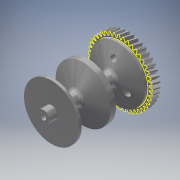
# Autodesk Inventor part: Spur Gear22
Saved by Autodesk Inventor 2019 (Build 230136000, 136)
## iProperties
Created: 2020-07-29
Part Number: Spur Gear22
Material: Steel
Document SubType Name: Modeling
Designer: Ian
Categories: <?xml version="1.0" encoding="UTF-16"?> <MemberInstance><Categories><FamilyTemplate><FamilyTemplateParameter ValueType="xs:double" Id="1" ObjectReferenceKey="da_z" ObjectType="kUserParameterObject"/><FamilyTemplateParameter ValueType="xs:double" Id="2" ObjectReferenceKey="da_b" ObjectType="kUserParameterObject"/><FamilyTemplateParameter ValueType="xs:double" Id="3" ObjectReferenceKey="da_beta" ObjectType="kUserParameterObject"/><FamilyTemplateParameter ValueType="xs:double" Id="4" ObjectReferenceKey="da_da" ObjectType="kUserParameterObject"/><FamilyTemplateParameter ValueType="xs:double" Id="5" ObjectReferenceKey="da_aw" ObjectType="kUserParameterObject"/><FamilyTemplateParameter ValueType="xs:string" Id="6" ObjectReferenceKey="EAIAABAAAACIAQAAAAAAAIAAAAAAAAAA" ObjectType="83910656" SubObjectId="SurfaceGeometry"/></FamilyTemplate><ParamToTemplateMap><ParamToTemplate CategoryParameter="//CategoryParameter[@InternalName='046C89C9-8512-4d59-83FE-43B91F4F132A']" TemplateParameter="1"/><ParamToTemplate CategoryParameter="//CategoryParameter[@InternalName='2552DF32-E462-4b46-AEBF-C6C7768E72AC']" TemplateParameter="2"/><ParamToTemplate CategoryParameter="//CategoryParameter[@InternalName='C9EE641D-15FC-4fae-A226-E94C4372FDD7']" TemplateParameter="3"/><ParamToTemplate><ParamToTemplate CategoryParameter="//CategoryParameter[@InternalName='00B6519A-459B-49c7-AD84-2E56D39A5744']" ConstantValue="0.281867"/></ParamToTemplate><ParamToTemplate><ParamToTemplate CategoryParameter="//CategoryParameter[@InternalName='04B31F0E-C7A6-4894-AA32-9629BEFACF47']" ConstantValue="1.000000"/></ParamToTemplate><ParamToTemplate><ParamToTemplate CategoryParameter="//CategoryParameter[@InternalName='43CBEC2E-7847-49e7-A936-2F7889FCB2D9']" ConstantValue="0.250000"/></ParamToTemplate><ParamToTemplate><ParamToTemplate CategoryParameter="//CategoryParameter[@InternalName='B1EFC894-105D-4ebd-86BF-FA20ED196853']" ConstantValue="0.350000"/></ParamToTemplate><ParamToTemplate><ParamToTemplate CategoryParameter="//CategoryParameter[@InternalName='51175063-3D10-4879-93E8-6246FE8B403D']" ConstantValue="2060000000.000000"/></ParamToTemplate><ParamToTemplate><ParamToTemplate CategoryParameter="//CategoryParameter[@InternalName='A3A52E27-4454-46a9-B0BD-C932399B70AF']" ConstantValue="0.300000"/></ParamToTemplate><ParamToTemplate><ParamToTemplate CategoryParameter="//CategoryParameter[@InternalName='91B76062-C214-41d9-B1B9-14D2AB99603D']" ConstantValue="0.050000"/></ParamToTemplate><ParamToTemplate><ParamToTemplate CategoryParameter="//CategoryParameter[@InternalName='374E806E-8B8A-4dda-A9AA-1039D6500AD2']" ConstantValue="20.000000"/></ParamToTemplate><ParamToTemplate><ParamToTemplate CategoryParameter="//CategoryParameter[@InternalName='2D373A89-B862-43d6-8D0B-0CBF12AB9F6C']" ConstantValue="0.349066"/></ParamToTemplate><ParamToTemplate CategoryParameter="//CategoryParameter[@InternalName='37777632-D6A2-4fac-9D53-DB8ACD95C989']" TemplateParameter="4"/><ParamToTemplate CategoryParameter="//CategoryParameter[@InternalName='FD1017F1-B727-4f7e-9707-0F86F1FF9423']" TemplateParameter="5"/><ParamToTemplate><ParamToTemplate CategoryParameter="//CategoryParameter[@InternalName='9E1B4470-B2D3-4ff1-B813-535BB4CDF51A']" ConstantValue="3520000.000000"/></ParamToTemplate><ParamToTemplate><ParamToTemplate CategoryParameter="//CategoryParameter[@InternalName='F8452263-BFF6-458c-9FB1-07C4B99E95CD']" ConstantValue="11400000.000000"/></ParamToTemplate><ParamToTemplate><ParamToTemplate CategoryParameter="//CategoryParameter[@InternalName='3E3BB259-FD49-497f-8171-6EBC954A3479']" ConstantValue="2.000000"/></ParamToTemplate><ParamToTemplate CategoryParameter="//CategoryParameter[@InternalName='27C3BAF2-7550-4e4b-AE2C-0DB134B7D9B7']" TemplateParameter="6"/></ParamToTemplateMap><Category DisplayName="Gear" InternalName="DC85795E-93AB-48d5-8EEE-5A27447B64BD" Mnemonic="Gear"><CategoryParameter DisplayName="z" InternalName="046C89C9-8512-4d59-83FE-43B91F4F132A" Mnemonic="z"/><CategoryParameter DisplayName="b" InternalName="2552DF32-E462-4b46-AEBF-C6C7768E72AC" Mnemonic="b"/><CategoryParameter DisplayName="||b|" InternalName="C9EE641D-15FC-4fae-A226-E94C4372FDD7" Mnemonic="beta"/><CategoryParameter DisplayName="x" InternalName="00B6519A-459B-49c7-AD84-2E56D39A5744" Mnemonic="x"/><CategoryParameter DisplayName="a*" InternalName="04B31F0E-C7A6-4894-AA32-9629BEFACF47" Mnemonic="a"/><CategoryParameter DisplayName="c*" InternalName="43CBEC2E-7847-49e7-A936-2F7889FCB2D9" Mnemonic="c"/><CategoryParameter DisplayName="r|.f|*" InternalName="B1EFC894-105D-4ebd-86BF-FA20ED196853" Mnemonic="rf"/><CategoryParameter DisplayName="E" InternalName="51175063-3D10-4879-93E8-6246FE8B403D" Mnemonic="E"/><CategoryParameter DisplayName="||m|" InternalName="A3A52E27-4454-46a9-B0BD-C932399B70AF" Mnemonic="mi"/><Category DisplayName="SpurGear" InternalName="26C5A22E-A91E-4dfd-A3B3-23CCAFAE1764" Mnemonic="SpurGear"><CategoryParameter DisplayName="m" InternalName="91B76062-C214-41d9-B1B9-14D2AB99603D" Mnemonic="m"/><CategoryParameter DisplayName="P" InternalName="374E806E-8B8A-4dda-A9AA-1039D6500AD2" Mnemonic="PP"/><CategoryParameter DisplayName="||a|" InternalName="2D373A89-B862-43d6-8D0B-0CBF12AB9F6C" Mnemonic="alpha"/><CategoryParameter DisplayName="d|.a|" InternalName="37777632-D6A2-4fac-9D53-DB8ACD95C989" Mnemonic="da"/><CategoryParameter DisplayName="a|.w|" InternalName="FD1017F1-B727-4f7e-9707-0F86F1FF9423" Mnemonic="aw"/><CategoryParameter DisplayName="||s||.Flim|" InternalName="9E1B4470-B2D3-4ff1-B813-535BB4CDF51A" Mnemonic="sFlim"/><CategoryParameter DisplayName="||s||.Hlim|" InternalName="F8452263-BFF6-458c-9FB1-07C4B99E95CD" Mnemonic="sHlim"/><CategoryParameter DisplayName="type" InternalName="3E3BB259-FD49-497f-8171-6EBC954A3479" Mnemonic="type"/><CategoryParameter DisplayName="PitchDiameter" InternalName="27C3BAF2-7550-4e4b-AE2C-0DB134B7D9B7" Mnemonic="IDS_PITCHDIAM"/></Category></Category></Categories></MemberInstance>
Density: 1 g/cm^3
Appearance: Steel
CustomPartVersion: 1
Author: Ian
Autodesk Inventor part; units mm, degrees
sketch "Sketch1" plane through (0, 0, 0) normal (0, 0, 1) x (1, 0, 0)
  circle A0 centre (0, 0) radius 11.6271
  dimension "d0" = 23.2542
  constraints: 1 centre point
  measures "d0" diameter of A0
extrude "Extrusion1" add sketch "Sketch1" along normal blind 3
ref_plane "Work Plane2" through (0, 0, 1.5) normal (0, 0, 1) x (1, 0, 0)
sketch "Sketch2" plane through (0, 0, 0) normal (0, 0, -1) x (-1, 0, 0)
  circle A0 centre (0, 0) radius 11.6271 projected
  circle A1 centre (0, 0) radius 11.0808
  dimension "d3" = 22.1615
  constraints: 1 centre point, 1 coincident
  measures "d3" diameter of A1
surface extrude "Pitch Diameter" sketch "Sketch2" against normal through all shown no curves A1
ref_plane "Work Plane8" through (0, 0, 0) normal (0.9973323, 0.0729953, 0) x (0, 0, 1)
ref_plane "Work Plane9" through (0, 0, 0) normal (1, 0, 0) x (0, 1, 0)
spur gear teeth "Spur Gear" teeth 43 pitch diameter 21.9803 tip diameter 23.2543 root diameter 21.0122 face width 3 helix angle 12 hand right start plane through (0, 0, 0) normal (0, 0, -1) x (-1, 0, 0)
sketch "Sketch3" plane through (0, 0, 0) normal (1, 0, 0) x (0, 1, 0)
  line L0 (-10, 3) -> (-10, 28) projected
  line L1 (10, 28) -> (10, 3) projected
  line L2 (-10, 28) -> (10, 28) projected
  line L3 (10, 3) -> (-10, 3) projected
  line L4 (-10, 3) -> (-10, 4)
  line L5 (-10, 4) -> (-2.25, 6.8208)
  line L6 (0, -35.2538) -> (0, 68.4313) projected
  line L7 (-2.25, 3) -> (-2.25, 28)
  line L8 (-10, 28) -> (-10, 27)
  line L9 (-10, 27) -> (-2.25, 24.1792)
  line L10 (-10, 15.5) -> (-5.6858, 15.5)
  line L11 (-10, 15.5) -> (-10, 14.5)
  line L12 (-10, 14.5) -> (-2.25, 11.6792)
  line L13 (-10, 15.5) -> (-10, 16.5)
  line L14 (-10, 16.5) -> (-2.25, 19.3208)
  point P0 (0, 0)
  dimension "d49" = 1
  dimension "d50" = 110
  dimension "d53" = 2.25
  dimension "d55" = 1
  dimension "d56" = 110
  dimension "d57" = 1
  dimension "d58" = 110
  dimension "d59" = 1
  dimension "d60" = 110
  constraints: 20 end point, 10 point on line, 2 midpoint, 1 horizontal, 1 parallel
  measures "d49" distance of L0.start L4.end
  measures "d50" angle of L4 L5
  measures "d53" distance between parallel lines of L6 L7
  measures "d55" distance of L0.end L8.end
  measures "d56" angle of L9 L8
  measures "d57" distance of L10.start L11.end
  measures "d58" angle of L12 L11
  measures "d59" distance of L10.start L13.end
  measures "d60" angle of L13 L14
revolve "Revolution1" add sketch "Sketch3" angle 360 about axis through (0, 0, -35.2538) along (0, 0, 1) contours L0 L5 L7 L3 | L0 L14 L7 L12 | L7 L9 L0 L2
sketch "Sketch4" plane through (0, 0, 3) normal (0, 0, 1) x (1, 0, 0)
  circle A0 centre (0, 0) radius 2.25 projected
  point P0 (0, 0)
extrude "Extrusion2" add sketch "Sketch4" along normal blind 28
fillet "Fillet1" radius 1.5 8 edges at (-1.591, 1.591, 6.8208) (1.591, -1.591, 6.8208) (1.591, -1.591, 11.6792) (-1.591, 1.591, 11.6792) (-1.591, 1.591, 19.3208) (1.591, -1.591, 19.3208) (1.591, -1.591, 24.1792) (-1.591, 1.591, 24.1792)
sketch "Sketch5" plane through (0, 0, 0) normal (0, 0, -1) x (-1, 0, 0)
  circle A0 centre (0, 0) radius 2.5
  dimension "d65" = 5
  constraints: 1 centre point, 1 coincident
  measures "d65" diameter of A0
extrude "Extrusion3" add sketch "Sketch5" along normal blind 3
sketch "Sketch7" plane through (0, 0, 3) normal (0, 0, 1) x (1, 0, 0)
  circle A0 centre (0, 0) radius 10 projected
  arc A1 (-3.7897, 10.9922) -> (-4.1886, 10.8465) centre (0, 0) ccw projected
  arc A2 (-5.3498, 10.3233) -> (-5.7232, 10.121) centre (0, 0) ccw projected
  arc A3 (-6.7958, 9.4343) -> (-7.1359, 9.1799) centre (0, 0) ccw projected
  arc A4 (-8.0971, 8.3443) -> (-8.3964, 8.043) centre (0, 0) ccw projected
  arc A5 (-9.2257, 7.0765) -> (-9.478, 6.7348) centre (0, 0) ccw projected
  arc A6 (-10.1577, 5.6578) -> (-10.3576, 5.283) centre (0, 0) ccw projected
  arc A7 (-10.8733, 4.1185) -> (-11.0164, 3.7186) centre (0, 0) ccw projected
  arc A8 (-11.3571, 2.4915) -> (-11.4405, 2.075) centre (0, 0) ccw projected
  arc A9 (-11.5988, 0.8113) -> (-11.6207, 0.3872) centre (0, 0) ccw projected
  arc A10 (-11.5933, -0.8861) -> (-11.5532, -1.309) centre (0, 0) ccw projected
  arc A11 (-11.3407, -2.5647) -> (-11.2395, -2.9772) centre (0, 0) ccw projected
  arc A12 (-10.8465, -4.1886) -> (-10.6863, -4.5819) centre (0, 0) ccw projected
  arc A13 (-10.121, -5.7232) -> (-9.9052, -6.089) centre (0, 0) ccw projected
  arc A14 (-9.1799, -7.1359) -> (-8.9131, -7.4664) centre (0, 0) ccw projected
  arc A15 (-8.043, -8.3964) -> (-7.731, -8.6846) centre (0, 0) ccw projected
  arc A16 (-6.7348, -9.478) -> (-6.3842, -9.7176) centre (0, 0) ccw projected
  arc A17 (-5.283, -10.3576) -> (-4.9012, -10.5436) centre (0, 0) ccw projected
  arc A18 (-3.7186, -11.0164) -> (-3.3138, -11.1449) centre (0, 0) ccw projected
  arc A19 (-2.075, -11.4405) -> (-1.6558, -11.5086) centre (0, 0) ccw projected
  arc A20 (-0.3872, -11.6207) -> (0.0375, -11.6271) centre (0, 0) ccw projected
  arc A21 (1.309, -11.5532) -> (1.73, -11.4977) centre (0, 0) ccw projected
  arc A22 (2.9772, -11.2395) -> (3.3857, -11.1233) centre (0, 0) ccw projected
  arc A23 (4.5819, -10.6863) -> (4.9692, -10.5118) centre (0, 0) ccw projected
  arc A24 (6.089, -9.9052) -> (6.4467, -9.6762) centre (0, 0) ccw projected
  arc A25 (7.4664, -8.9131) -> (7.7869, -8.6345) centre (0, 0) ccw projected
  arc A26 (8.6846, -7.731) -> (8.9611, -7.4087) centre (0, 0) ccw projected
  arc A27 (9.7176, -6.3842) -> (9.9443, -6.025) centre (0, 0) ccw projected
  arc A28 (10.5436, -4.9012) -> (10.7156, -4.5129) centre (0, 0) ccw projected
  arc A29 (11.1449, -3.3138) -> (11.2585, -2.9046) centre (0, 0) ccw projected
  arc A30 (11.5086, -1.6558) -> (11.5614, -1.2344) centre (0, 0) ccw projected
  arc A31 (11.6271, 0.0375) -> (11.6179, 0.4621) centre (0, 0) ccw projected
  arc A32 (11.4977, 1.73) -> (11.4268, 2.1488) centre (0, 0) ccw projected
  arc A33 (11.1233, 3.3857) -> (10.9922, 3.7897) centre (0, 0) ccw projected
  arc A34 (10.5118, 4.9692) -> (10.3233, 5.3498) centre (0, 0) ccw projected
  arc A35 (9.6762, 6.4467) -> (9.4343, 6.7958) centre (0, 0) ccw projected
  arc A36 (8.6345, 7.7869) -> (8.3443, 8.0971) centre (0, 0) ccw projected
  arc A37 (7.4087, 8.9611) -> (7.0765, 9.2257) centre (0, 0) ccw projected
  arc A38 (6.025, 9.9443) -> (5.6578, 10.1577) centre (0, 0) ccw projected
  arc A39 (4.5129, 10.7156) -> (4.1185, 10.8733) centre (0, 0) ccw projected
  arc A40 (2.9046, 11.2585) -> (2.4915, 11.3571) centre (0, 0) ccw projected
  arc A41 (1.2344, 11.5614) -> (0.8113, 11.5988) centre (0, 0) ccw projected
  arc A42 (-0.4621, 11.6179) -> (-0.8861, 11.5933) centre (0, 0) ccw projected
  arc A43 (-2.1488, 11.4268) -> (-2.5647, 11.3407) centre (0, 0) ccw projected
  constraints: 129 other
sketch "Sketch8" plane through (0, 0, 0) normal (0, 0, -1) x (-1, 0, 0)
  line L0 (0, 5.7735) -> (5, -2.8868)
  line L1 (5, -2.8868) -> (-5, -2.8868)
  line L2 (-5, -2.8868) -> (0, 5.7735)
  circle A0 centre (0, 5.7735) radius 1.05
  circle A1 centre (5, -2.8868) radius 1.05
  circle A2 centre (-5, -2.8868) radius 1.05
  point P0 (0, 0)
  point P1 (0, 0)
  dimension "d69" = 10
  dimension "d70" = 2.1
  dimension "d71" = 2.1
  dimension "d72" = 2.1
  constraints: 6 end point, 4 coincident, 3 centre point, 1 horizontal, 7 other
  measures "d69" distance of L0.end L1.end
  measures "d70" diameter of A0
  measures "d71" diameter of A1
  measures "d72" diameter of A2
extrude "Extrusion4" cut sketch "Sketch8" against normal up to surface contours L2 A0 L0 | L0 A0 L2 | A1 L1 L0 | L0 L1 A1 | A2 L1 L2 | L2 L1 A2
sketch "Sketch9" plane through (0, 0, -3) normal (0, 0, -1) x (-1, 0, 0)
  circle A0 centre (0, 0) radius 1.05
  dimension "d75" = 2.1
  constraints: 1 centre point, 1 coincident
  measures "d75" diameter of A0
extrude "Extrusion5" cut sketch "Sketch9" along normal through all both and the other way through all
sketch "Sketch10" plane through (0, 0, -3) normal (0, 0, -1) x (-1, 0, 0)
  circle A0 centre (0, 0) radius 1.05 projected
  circle A1 centre (0, 0) radius 2.5 projected
  circle A2 centre (0, 0) radius 2.25
  dimension "d78" = 4.5
  constraints: 1 centre point, 1 coincident
  measures "d78" diameter of A2
extrude "Extrusion6" cut sketch "Sketch10" against normal up to surface (3 mm away) contours A1
equation "\"d0\" = da_da"
equation "\"d1\" = da_b"
equation "\"d3\" = da_dw"
equation "\"d16\" = da_aw"
equation "\"d43\" = da_aw"
equation "\"d46\" = da_aw"
equation "\"da_da\" = 23.254253"
equation "\"da_b\" = 3"
equation "\"da_dw\" = 22.161538"
equation "\"da_aw\" = 16.75"
body "Solid1"
body "Srf1"
